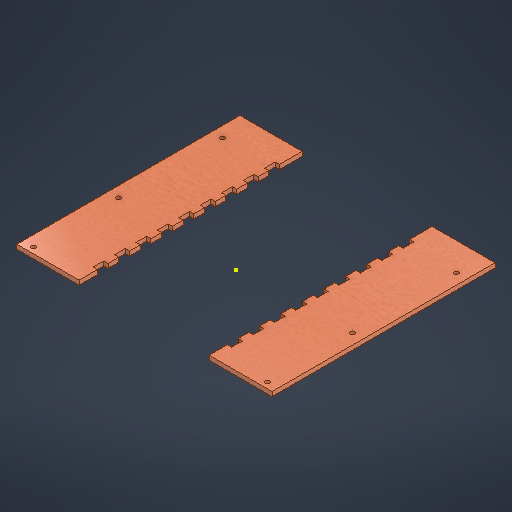
# Autodesk Inventor part: стульчак
Saved by Autodesk Inventor 2025 (Build 290162000, 162)
## iProperties
Created: 2025-01-28
Part Number: стульчак
Material: Древесина (орех)
Document SubType Name: Modeling
Designer: GameHD
Density: 0.55 g/cm^3
Appearance: Орех — натуральный — полированный
Author: GameHD
Autodesk Inventor part; units mm, degrees
ref_plane "YZ Plane" through (0, 0, 0) normal (1, 0, 0) x (0, 1, 0)
ref_plane "XZ Plane" through (0, 0, 0) normal (0, 1, 0) x (-1, 0, 0)
ref_plane "XY Plane" through (0, 0, 0) normal (0, 0, 1) x (1, 0, 0)
sketch "Эскиз1" plane through (0, 0, 0) normal (0, 1, 0) x (-1, 0, 0)
  line L0 (-115, 123) -> (115, 123)
  line L1 (115, 123) -> (115, -123)
  line L2 (115, -123) -> (-115, -123)
  line L3 (-115, -123) -> (-115, 123)
  line L4 (-115, 123) -> (115, -123) construction
  line L5 (115, 123) -> (-115, -123) construction
  point P0 (0, 0)
  dimension "d0" = 230
  dimension "d1" = 246
  constraints: 12 end point, 2 midpoint, 2 parallel, 1 horizontal, 1 perpendicular
  measures "d0" distance of L1.end L2.end
  measures "d1" distance of L0.end L1.end
extrude "Выдавливание1" add sketch "Эскиз1" along normal blind 4
sketch "Эскиз2" plane through (0, 0, 0) normal (0, -1, 0) x (1, 0, 0)
  line L0 (-65.9289, -30.8784) -> (-65.9289, 53.4389) projected
  line L1 (65.9289, -33.6328) -> (65.9289, 50.6846) projected
  line L2 (115, -123) -> (-115, -123) projected
  line L3 (-115, 123) -> (115, 123) projected
  line L4 (-115, -123) -> (-61, -123)
  line L5 (-61, -123) -> (-61, 123)
  line L6 (-61, 123) -> (-115, 123)
  line L7 (-115, 123) -> (-115, -123)
  line L8 (114.3, -123) -> (60.3, -123)
  line L9 (60.3, -123) -> (60.3, 123)
  line L10 (60.3, 123) -> (114.3, 123)
  line L11 (114.3, 123) -> (114.3, -123)
  line L12 (21.8052, 115.9865) -> (21.8052, 75.1678) projected
  line L13 (60.3, 123) -> (-61.2, 123)
  line L14 (-61.2, 123) -> (-61.2, 68)
  line L15 (-61.2, 68) -> (60.3, 68)
  line L16 (60.3, 68) -> (60.3, 123)
  line L17 (115, -123) -> (-115, -123) projected
  line L18 (115, 123) -> (115, -123) projected
  line L19 (-115, 123) -> (115, 123) projected
  line L20 (-115, -123) -> (-115, 123) projected
  point P0 (0, 0)
  point P1 (-61, 68)
  point P2 (60.3, -123)
  dimension "d4" = 54
  dimension "d5" = 54
  dimension "d7" = 55
  dimension "d90" = 121.5
  constraints: 24 end point, 6 parallel, 3 horizontal, 3 perpendicular, 3 point on line, 1 vertical
  measures "d4" distance of L6.end L5.end
  measures "d5" distance of L9.end L10.end
  measures "d7" distance of L14.end L13.end
  measures "d90" distance of L14.end L15.end
extrude "Выдавливание2" cut sketch "Эскиз2" against normal blind 4 contours L2 L5 L15 L9 | L15 L5 L3 L9
sketch "Эскиз3" plane through (0, 0, 0) normal (0, -1, 0) x (1, 0, 0)
  point P0 (0, 0)
sketch "Эскиз4" plane through (0, 0, 0) normal (0, -1, 0) x (1, 0, 0)
  point P0 (0, 0)
sketch "Эскиз5" plane through (0, 0, 0) normal (0, -1, 0) x (1, 0, 0)
  line L0 (-61, 123) -> (-61, -123) projected
  line L1 (-61, 68) -> (-65, 68)
  line L2 (-65, 68) -> (-65, 58)
  line L3 (-65, 58) -> (-61, 58)
  line L4 (-61, 58) -> (-61, 68)
  line L5 (-61, 78) -> (-65, 78)
  line L6 (-65, 78) -> (-65, 68)
  line L7 (-65, 68) -> (-61, 68)
  line L8 (-61, 68) -> (-61, 78)
  line L9 (-61, 68) -> (-65, 68)
  line L10 (-65, 68) -> (-65, 58)
  line L11 (-65, 58) -> (-61, 58)
  line L12 (-61, 58) -> (-61, 68)
  line L13 (-61, 58) -> (-65, 58)
  line L14 (-65, 58) -> (-65, 48)
  line L15 (-65, 48) -> (-61, 48)
  line L16 (-61, 48) -> (-61, 58)
  line L17 (-61, 48) -> (-65, 48)
  line L18 (-65, 48) -> (-65, 38)
  line L19 (-65, 38) -> (-61, 38)
  line L20 (-61, 38) -> (-61, 48)
  line L21 (-61, 38) -> (-65, 38)
  line L22 (-65, 38) -> (-65, 28)
  line L23 (-65, 28) -> (-61, 28)
  line L24 (-61, 28) -> (-61, 38)
  line L25 (-61, 28) -> (-65, 28)
  line L26 (-65, 28) -> (-65, 18)
  line L27 (-65, 18) -> (-61, 18)
  line L28 (-61, 18) -> (-61, 28)
  line L29 (-61, 18) -> (-65, 18)
  line L30 (-65, 18) -> (-65, 8)
  line L31 (-65, 8) -> (-61, 8)
  line L32 (-61, 8) -> (-61, 18)
  line L33 (-61, 8) -> (-65, 8)
  line L34 (-65, 8) -> (-65, -2)
  line L35 (-65, -2) -> (-61, -2)
  line L36 (-61, -2) -> (-61, 8)
  line L37 (-61, -2) -> (-65, -2)
  line L38 (-65, -2) -> (-65, -12)
  line L39 (-65, -12) -> (-61, -12)
  line L40 (-61, -12) -> (-61, -2)
  line L41 (-61, -12) -> (-65, -12)
  line L42 (-65, -12) -> (-65, -22)
  line L43 (-65, -22) -> (-61, -22)
  line L44 (-61, -22) -> (-61, -12)
  line L45 (-61, -22) -> (-65, -22)
  line L46 (-65, -22) -> (-65, -32)
  line L47 (-65, -32) -> (-61, -32)
  line L48 (-61, -32) -> (-61, -22)
  line L49 (-61, -32) -> (-65, -32)
  line L50 (-65, -32) -> (-65, -42)
  line L51 (-65, -42) -> (-61, -42)
  line L52 (-61, -42) -> (-61, -32)
  line L53 (-61, -42) -> (-65, -42)
  line L54 (-65, -42) -> (-65, -52)
  line L55 (-65, -52) -> (-61, -52)
  line L56 (-61, -52) -> (-61, -42)
  line L57 (-61, -52) -> (-65, -52)
  line L58 (-65, -52) -> (-65, -62)
  line L59 (-65, -62) -> (-61, -62)
  line L60 (-61, -62) -> (-61, -52)
  line L61 (-61, -62) -> (-65, -62)
  line L62 (-65, -62) -> (-65, -72)
  line L63 (-65, -72) -> (-61, -72)
  line L64 (-61, -72) -> (-61, -62)
  line L65 (-61, -72) -> (-65, -72)
  line L66 (-65, -72) -> (-65, -82)
  line L67 (-65, -82) -> (-61, -82)
  line L68 (-61, -82) -> (-61, -72)
  line L69 (-61, -82) -> (-65, -82)
  line L70 (-65, -82) -> (-65, -92)
  line L71 (-65, -92) -> (-61, -92)
  line L72 (-61, -92) -> (-61, -82)
  line L73 (-61, -92) -> (-65, -92)
  line L74 (-65, -92) -> (-65, -102)
  line L75 (-65, -102) -> (-61, -102)
  line L76 (-61, -102) -> (-61, -92)
  line L77 (-61, -102) -> (-65, -102)
  line L78 (-65, -102) -> (-65, -112)
  line L79 (-61, -112) -> (-61, -102)
  line L80 (-0.35, 88) -> (-0.35, -60.325)
  line L81 (60.3, 68) -> (60.3, -123)
  line L82 (60.3, 68) -> (64.3, 68)
  line L83 (64.3, 68) -> (64.3, 58)
  line L84 (64.3, 58) -> (60.3, 58)
  line L85 (60.3, 58) -> (60.3, 68)
  line L86 (64.3, 68) -> (60.3, 68)
  line L87 (64.3, 78) -> (64.3, 68)
  line L88 (60.3, 78) -> (64.3, 78)
  line L89 (60.3, 68) -> (60.3, 78)
  line L90 (64.3, 58) -> (60.3, 58)
  line L91 (64.3, 68) -> (64.3, 58)
  line L92 (60.3, 68) -> (64.3, 68)
  line L93 (60.3, 58) -> (60.3, 68)
  line L94 (64.3, 48) -> (60.3, 48)
  line L95 (64.3, 58) -> (64.3, 48)
  line L96 (60.3, 58) -> (64.3, 58)
  line L97 (60.3, 48) -> (60.3, 58)
  line L98 (64.3, 38) -> (60.3, 38)
  line L99 (64.3, 48) -> (64.3, 38)
  line L100 (60.3, 48) -> (64.3, 48)
  line L101 (60.3, 38) -> (60.3, 48)
  line L102 (64.3, 28) -> (60.3, 28)
  line L103 (64.3, 38) -> (64.3, 28)
  line L104 (60.3, 38) -> (64.3, 38)
  line L105 (60.3, 28) -> (60.3, 38)
  line L106 (64.3, 18) -> (60.3, 18)
  line L107 (64.3, 28) -> (64.3, 18)
  line L108 (60.3, 28) -> (64.3, 28)
  line L109 (60.3, 18) -> (60.3, 28)
  line L110 (64.3, 8) -> (60.3, 8)
  line L111 (64.3, 18) -> (64.3, 8)
  line L112 (60.3, 18) -> (64.3, 18)
  line L113 (60.3, 8) -> (60.3, 18)
  line L114 (64.3, -2) -> (60.3, -2)
  line L115 (64.3, 8) -> (64.3, -2)
  line L116 (60.3, 8) -> (64.3, 8)
  line L117 (60.3, -2) -> (60.3, 8)
  line L118 (64.3, -12) -> (60.3, -12)
  line L119 (64.3, -2) -> (64.3, -12)
  line L120 (60.3, -2) -> (64.3, -2)
  line L121 (60.3, -12) -> (60.3, -2)
  line L122 (64.3, -22) -> (60.3, -22)
  line L123 (64.3, -12) -> (64.3, -22)
  line L124 (60.3, -12) -> (64.3, -12)
  line L125 (60.3, -22) -> (60.3, -12)
  line L126 (64.3, -32) -> (60.3, -32)
  line L127 (64.3, -22) -> (64.3, -32)
  line L128 (60.3, -22) -> (64.3, -22)
  line L129 (60.3, -32) -> (60.3, -22)
  line L130 (64.3, -42) -> (60.3, -42)
  line L131 (64.3, -32) -> (64.3, -42)
  line L132 (60.3, -32) -> (64.3, -32)
  line L133 (60.3, -42) -> (60.3, -32)
  line L134 (64.3, -52) -> (60.3, -52)
  line L135 (64.3, -42) -> (64.3, -52)
  line L136 (60.3, -42) -> (64.3, -42)
  line L137 (60.3, -52) -> (60.3, -42)
  line L138 (64.3, -62) -> (60.3, -62)
  line L139 (64.3, -52) -> (64.3, -62)
  line L140 (60.3, -52) -> (64.3, -52)
  line L141 (60.3, -62) -> (60.3, -52)
  line L142 (64.3, -72) -> (60.3, -72)
  line L143 (64.3, -62) -> (64.3, -72)
  line L144 (60.3, -62) -> (64.3, -62)
  line L145 (60.3, -72) -> (60.3, -62)
  line L146 (64.3, -82) -> (60.3, -82)
  line L147 (64.3, -72) -> (64.3, -82)
  line L148 (60.3, -72) -> (64.3, -72)
  line L149 (60.3, -82) -> (60.3, -72)
  line L150 (64.3, -92) -> (60.3, -92)
  line L151 (64.3, -82) -> (64.3, -92)
  line L152 (60.3, -82) -> (64.3, -82)
  line L153 (60.3, -92) -> (60.3, -82)
  line L154 (64.3, -102) -> (60.3, -102)
  line L155 (64.3, -92) -> (64.3, -102)
  line L156 (60.3, -92) -> (64.3, -92)
  line L157 (60.3, -102) -> (60.3, -92)
  line L158 (64.3, -102) -> (64.3, -112)
  line L159 (60.3, -102) -> (64.3, -102)
  line L160 (60.3, -112) -> (60.3, -102)
  point P0 (0, 0)
  point P1 (-61, -102)
  point P2 (-61, -92)
  point P3 (-61, -82)
  point P4 (-61, -72)
  point P5 (-61, -62)
  point P6 (-61, -52)
  point P7 (-61, -42)
  point P8 (-61, -32)
  point P9 (-61, -22)
  point P10 (-61, -12)
  point P11 (-61, -2)
  point P12 (-61, 8)
  point P13 (-61, 18)
  point P14 (-61, 28)
  point P15 (-61, 38)
  point P16 (-61, 48)
  point P17 (60.3, -92)
  point P18 (60.3, -102)
  point P19 (60.3, -72)
  point P20 (60.3, -82)
  point P21 (60.3, -52)
  point P22 (60.3, -62)
  point P23 (60.3, -32)
  point P24 (60.3, -42)
  point P25 (-61, -12)
  point P26 (-61, 8)
  dimension "d10" = 4
  dimension "d11" = 10
  dimension "d12" = 4
  dimension "d13" = 10
  dimension "d14" = 4
  dimension "d15" = 10
  dimension "d16" = 4
  dimension "d17" = 10
  dimension "d18" = 4
  dimension "d19" = 10
  dimension "d20" = 4
  dimension "d21" = 10
  dimension "d22" = 4
  dimension "d23" = 10
  dimension "d24" = 4
  dimension "d25" = 10
  dimension "d26" = 4
  dimension "d27" = 10
  dimension "d28" = 4
  dimension "d29" = 10
  dimension "d30" = 4
  dimension "d31" = 10
  dimension "d32" = 4
  dimension "d33" = 10
  dimension "d34" = 4
  dimension "d35" = 10
  dimension "d36" = 4
  dimension "d37" = 10
  dimension "d38" = 4
  dimension "d39" = 10
  dimension "d40" = 4
  dimension "d41" = 10
  dimension "d42" = 4
  dimension "d43" = 10
  dimension "d44" = 4
  dimension "d45" = 10
  dimension "d46" = 4
  dimension "d47" = 10
  dimension "d49" = 10
  constraints: 320 end point, 39 parallel, 20 horizontal, 20 perpendicular, 4 symmetric about line, 1 vertical, 1 other
  measures "d10" distance of L3.end L2.end
  measures "d11" distance of L2.end L1.end
  measures "d12" distance of L7.end L7.start
  measures "d13" distance of L7.start L6.start
  measures "d14" distance of L11.end L11.start
  measures "d15" distance of L11.start L10.start
  measures "d16" distance of L15.end L15.start
  measures "d17" distance of L15.start L14.start
  measures "d18" distance of L19.end L19.start
  measures "d19" distance of L19.start L18.start
  measures "d20" distance of L23.end L23.start
  measures "d21" distance of L23.start L22.start
  measures "d22" distance of L27.end L27.start
  measures "d23" distance of L27.start L26.start
  measures "d24" distance of L31.end L31.start
  measures "d25" distance of L31.start L30.start
  measures "d26" distance of L35.end L35.start
  measures "d27" distance of L35.start L34.start
  measures "d28" distance of L39.end L39.start
  measures "d29" distance of L39.start L38.start
  measures "d30" distance of L43.end L43.start
  measures "d31" distance of L43.start L42.start
  measures "d32" distance of L47.end L47.start
  measures "d33" distance of L47.start L46.start
  measures "d34" distance of L51.end L51.start
  measures "d35" distance of L51.start L50.start
  measures "d36" distance of L55.end L55.start
  measures "d37" distance of L55.start L54.start
  measures "d38" distance of L59.end L59.start
  measures "d39" distance of L59.start L58.start
  measures "d40" distance of L63.end L63.start
  measures "d41" distance of L63.start L62.start
  measures "d42" distance of L67.end L67.start
  measures "d43" distance of L67.start L66.start
  measures "d44" distance of L71.end L71.start
  measures "d45" distance of L71.start L70.start
  measures "d46" distance of L75.end L75.start
  measures "d47" distance of L75.start L74.start
  measures "d49" distance of L78.end L78.start
extrude "Выдавливание3" cut sketch "Эскиз5" against normal blind 4 contours L0 L3 L2 L1 | L0 L19 L18 L15 | L0 L27 L26 L23 | L0 L35 L34 L31 | L0 L43 L42 L39 | L0 L51 L50 L47 | L0 L59 L58 L55 | L0 L67 L66 L63 | L0 L75 L74 L71 | L82 L83 L84 L81 | L94 L99 L98 L81 | L102 L107 L106 L81 | L110 L115 L114 L81 | L118 L123 L122 L81 | L126 L131 L130 L81 | L134 L139 L138 L81 | L142 L147 L146 L81 | L150 L155 L154 L81
sketch "Эскиз6" plane through (0, 0, 0) normal (0, -1, 0) x (1, 0, 0)
  line L0 (-115, -123) -> (-115, 123) projected
  line L1 (-115, 123) -> (-109, 123)
  line L2 (-115, 123) -> (115, 123) projected
  line L3 (-109, 123) -> (-109, -139.0315)
  circle A0 centre (-109, 79.375) radius 2.1
  circle A1 centre (-109, 0) radius 2.1
  circle A2 centre (-109, -96.8375) radius 2.1
  line L4 (0, 123) -> (0, -68.2625)
  circle A3 centre (109, 79.375) radius 2.1
  circle A4 centre (109, 0) radius 2.1
  circle A5 centre (109, -96.8375) radius 2.1
  line L5 (109, 123) -> (109, -139.0315)
  point P0 (0, 0)
  point P1 (-115, 0)
  dimension "d79" = 6
  dimension "d80" = 4.2
  dimension "d81" = 4.2
  dimension "d82" = 4.2
  dimension "d89" = 12
  constraints: 8 end point, 6 centre point, 5 symmetric about line, 3 point on line, 2 midpoint, 1 perpendicular, 1 vertical, 3 other
  measures "d79" distance of L0.end L1.end
  measures "d80" diameter of A0
  measures "d81" diameter of A1
  measures "d82" diameter of A2
  measures "d89" diameter of A1.centre point (-115, 0)
extrude "Выдавливание4" cut sketch "Эскиз6" against normal blind 4.2
sketch "Эскиз7" plane through (0, 0, 0) normal (0, -1, 0) x (1, 0, 0)
  line L0 (-115, 123) -> (-119, 123)
  line L1 (-119, 123) -> (-119, -123)
  line L2 (-119, -123) -> (-115, -123)
  line L3 (-115, -123) -> (-115, 123)
  line L4 (115, 123) -> (115, -123) projected
  line L5 (115, -123) -> (119, -123)
  line L6 (119, -123) -> (119, 123)
  line L7 (119, 123) -> (115, 123)
  line L8 (115, 123) -> (115, -123)
  point P0 (0, 0)
  dimension "d85" = 4
  dimension "d86" = 4
  constraints: 16 end point, 4 parallel, 2 horizontal, 2 perpendicular, 1 point on line
  measures "d85" distance of L2.end L1.end
  measures "d86" distance of L7.end L6.end
extrude "Выдавливание5" add sketch "Эскиз7" against normal up to surface (4 mm away)
sketch "Эскиз8" plane through (0, 0, 0) normal (0, -1, 0) x (1, 0, 0)
  point P0 (0, 0)
sketch "Эскиз9" plane through (0, 0, 0) normal (0, -1, 0) x (1, 0, 0)
  line L0 (119, 123) -> (-119, 123) projected
  line L1 (-119, 123) -> (-61, 123)
  line L2 (-61, 123) -> (-61, 85)
  line L3 (-61, 85) -> (-119, 85)
  line L4 (-119, 85) -> (-119, 123)
  line L5 (119, 123) -> (59, 123)
  line L6 (59, 123) -> (59, 85)
  line L7 (59, 85) -> (119, 85)
  line L8 (119, 85) -> (119, 123)
  point P0 (0, 0)
  point P1 (-81.9049, 71.7303)
  point P2 (-61, 123)
  dimension "d92" = 58
  dimension "d93" = 38
  dimension "d94" = 60
  dimension "d95" = 38
  constraints: 16 end point, 4 parallel, 2 horizontal, 2 perpendicular, 1 other
  measures "d92" distance of L2.end L3.end
  measures "d93" distance of L1.end L2.end
  measures "d94" distance of L7.end L6.end
  measures "d95" distance of L6.end L5.end
extrude "Выдавливание6" cut sketch "Эскиз9" against normal blind 10
equation "\"d52\" = d16"
